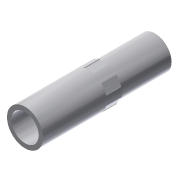
# Autodesk Inventor part: PP-06
Saved by Autodesk Inventor 2022 (Build 260148000, 148)
## iProperties
Created: 2008-09-23
Part Number: PP-06
Document SubType Name: Modeling
Designer: Mark Flayler
Mass: 0.223339 g
Surface Area: 6.17982 cm^2
Volume: 0.210697 cm^3
Density: 1.06 g/cm^3
Material: ABS Plastic
Description: SHAFT DISPENSER
Appearance: Smooth - White
Author: Mark Flayler
Autodesk Inventor part; units mm, degrees
ref_plane "YZ Plane" through (0, 0, 0) normal (1, 0, 0) x (0, 1, 0)
sketch "Sketch1" plane through (0, 0, 0) normal (0, 0, 1) x (1, 0, 0)
  line L0 (0, 0) -> (0, 20)
  line L1 (2.1, 0) -> (2.775, 0)
  line L2 (2.775, 0) -> (2.775, 12.2)
  line L3 (2.775, 12.2) -> (2.55, 12.2)
  line L4 (2.55, 12.2) -> (2.55, 20)
  line L5 (2.55, 20) -> (1.7, 20)
  line L6 (1.7, 20) -> (1.7, 17.8)
  line L7 (1.7, 17.8) -> (1.5, 17.8)
  line L8 (1.5, 17.8) -> (1.5, 14)
  line L9 (1.5, 14) -> (2.1, 14)
  line L10 (2.1, 14) -> (2.1, 0)
  dimension "d0" = 3.4
  dimension "d1" = 3
  dimension "d3" = 4.2
  dimension "d4" = 12.2
  dimension "d5" = 20
  dimension "d6" = 14
  dimension "d7" = 17.8
  dimension "d8" = 5.55
  dimension "d9" = 5.1
  constraints: 22 end point, 8 parallel, 2 horizontal alignment, 2 perpendicular, 1 vertical
  measures "d0" diameter of L6 L0
  measures "d1" diameter of L8 L0
  measures "d3" diameter of L10 L0
  measures "d4" distance from line of L0.start L3
  measures "d5" distance from line of L0.start L5
  measures "d6" distance from line of L0.start L9
  measures "d7" distance from line of L0.start L7
  measures "d8" diameter of L2 L0
  measures "d9" diameter of L4 L0
revolve "Revolution1" add sketch "Sketch1" angle 360 about axis through (0, 0, 0) along (0, 1, 0)
ref_plane "Work Plane1" through (0, 6.1, 2.775) normal (0, 0, 1) x (1, 0, 0)
sketch "Sketch2" plane through (0, 6.1, 2.775) normal (0, 0, 1) x (1, 0, 0)
  line L0 (-2.775, 6.1) -> (2.775, 6.1) projected
  line L1 (-2.775, -6.1) -> (2.775, -6.1) projected
  line L2 (-0.7265, 6.1) -> (0.7265, 6.1)
  line L3 (0.7265, 6.1) -> (0.7265, 3.7)
  line L4 (0.7265, 3.7) -> (-0.7265, 3.7)
  line L5 (-0.7265, 3.7) -> (-0.7265, 6.1)
  line L6 (0, -10.1) -> (0, 17.9) projected
  dimension "d12" = 9.8
  dimension "d13" = 1.453
  constraints: 8 end point, 2 parallel, 1 horizontal, 1 perpendicular, 1 point on line, 1 other
  measures "d12" distance between parallel lines of L4 L1
  measures "d13" distance between parallel lines of L3 L5
ref_plane "Work Plane2" through (0, 0, 2.6) normal (0, 0, 1) x (1, 0, 0)
extrude "Extrusion1" cut sketch "Sketch2" against normal up to surface (0.175 mm away)
pattern_circular "Circular Pattern1" count 6 over 360 about axis through (0, 6.1, 0) along (0, -1, 0) of "Extrusion1"
body "Solid1"
